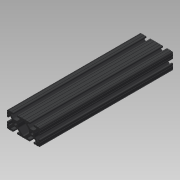
# Autodesk Inventor part: 1530
Saved by Autodesk Inventor 2013 (Build 170138000, 138)
## iProperties
Company: 80/20 Inc.
Created: 2014-04-23
Part Number: 1530
Material: Generic
Document SubType Name: Modeling
Density: 1 g/cm^3
Vendor: 80/20 Inc.
Engineer: Ross Bowman
Designer: Ross Bowman
Catalog Web Link: 8020.net
Material: 6105-T5 Aluminum
Author: Ross Bowman
Keywords: 80/20 , 8020 , T-Slot , Extrusion
Autodesk Inventor part; units mm, degrees
ref_plane "YZ Plane" through (0, 0, 0) normal (1, 0, 0) x (0, 1, 0)
ref_plane "XZ Plane" through (0, 0, 0) normal (0, 1, 0) x (-1, 0, 0)
ref_plane "XY Plane" through (0, 0, 0) normal (0, 0, 1) x (1, 0, 0)
sketch "Sketch1" plane through (0, 0, 0) normal (0, 0, 1) x (1, 0, 0)
  circle A0 centre (-19.05, 0) radius 3.3274
  circle A1 centre (19.05, 0) radius 3.3274
  arc A2 (0, -15.1131) -> (2.077, -14.2576) centre (0.0116, -12.1921) ccw
  arc A3 (-2.077, -14.2576) -> (0, -15.1131) centre (-0.0116, -12.1921) ccw
  line L0 (-10.9024, -5.4321) -> (-2.077, -14.2576)
  arc A4 (-12.2936, -2.0735) -> (-10.9024, -5.4321) centre (-7.5438, -2.0735) ccw
  line L1 (-12.2936, 2.0735) -> (-12.2936, -2.0735)
  arc A5 (-10.9024, 5.4321) -> (-12.2936, 2.0735) centre (-7.5438, 2.0735) ccw
  line L2 (-2.077, 14.2576) -> (-10.9024, 5.4321)
  arc A6 (0, 15.1131) -> (-2.077, 14.2576) centre (-0.0116, 12.1921) ccw
  arc A7 (2.077, 14.2576) -> (0, 15.1131) centre (0.0116, 12.1921) ccw
  line L3 (10.9024, 5.4321) -> (2.077, 14.2576)
  arc A8 (12.2936, 2.0735) -> (10.9024, 5.4321) centre (7.5438, 2.0735) ccw
  line L4 (12.2936, -2.0735) -> (12.2936, 2.0735)
  arc A9 (10.9024, -5.4321) -> (12.2936, -2.0735) centre (7.5438, -2.0735) ccw
  line L5 (2.077, -14.2576) -> (10.9024, -5.4321)
  arc A10 (8.9158, 13.5344) -> (9.1761, 12.9058) centre (9.8048, 13.5344) ccw
  line L6 (8.9158, 13.5344) -> (8.9158, 14.097)
  arc A11 (9.8048, 14.986) -> (8.9158, 14.097) centre (9.8048, 14.097) ccw
  line L7 (9.8048, 14.986) -> (13.4112, 14.986)
  arc A12 (13.4112, 14.986) -> (14.986, 16.5608) centre (13.4112, 16.5608) ccw
  line L8 (14.986, 16.5608) -> (14.986, 17.4968)
  arc A13 (14.986, 17.4968) -> (13.4328, 19.05) centre (13.4328, 17.4968) ccw
  line L9 (13.4328, 19.05) -> (10.9975, 19.05)
  arc A14 (9.4735, 19.05) -> (10.9975, 19.05) centre (10.2355, 19.05) ccw
  line L10 (9.4735, 19.05) -> (4.6451, 19.05)
  arc A15 (3.1211, 19.05) -> (4.6451, 19.05) centre (3.8831, 19.05) ccw
  line L11 (3.1211, 19.05) -> (-3.1211, 19.05)
  arc A16 (-4.6451, 19.05) -> (-3.1211, 19.05) centre (-3.8831, 19.05) ccw
  line L12 (-4.6451, 19.05) -> (-9.4735, 19.05)
  arc A17 (-10.9975, 19.05) -> (-9.4735, 19.05) centre (-10.2355, 19.05) ccw
  line L13 (-10.9975, 19.05) -> (-13.4328, 19.05)
  arc A18 (-13.4328, 19.05) -> (-14.986, 17.4968) centre (-13.4328, 17.4968) ccw
  line L14 (-14.986, 17.4968) -> (-14.986, 16.5608)
  arc A19 (-14.986, 16.5608) -> (-13.4112, 14.986) centre (-13.4112, 16.5608) ccw
  line L15 (-13.4112, 14.986) -> (-9.8048, 14.986)
  arc A20 (-8.9158, 14.097) -> (-9.8048, 14.986) centre (-9.8048, 14.097) ccw
  line L16 (-8.9158, 14.097) -> (-8.9158, 13.5344)
  arc A21 (-9.1761, 12.9058) -> (-8.9158, 13.5344) centre (-9.8048, 13.5344) ccw
  line L17 (-9.1761, 12.9058) -> (-13.8525, 8.2294)
  arc A22 (-17.2111, 6.8382) -> (-13.8525, 8.2294) centre (-17.2111, 11.588) ccw
  line L18 (-17.2111, 6.8382) -> (-20.8889, 6.8382)
  arc A23 (-24.2475, 8.2294) -> (-20.8889, 6.8382) centre (-20.8889, 11.588) ccw
  line L19 (-24.2475, 8.2294) -> (-28.9239, 12.9058)
  arc A24 (-29.1842, 13.5344) -> (-28.9239, 12.9058) centre (-28.2952, 13.5344) ccw
  line L20 (-29.1842, 13.5344) -> (-29.1842, 14.097)
  arc A25 (-28.2952, 14.986) -> (-29.1842, 14.097) centre (-28.2952, 14.097) ccw
  line L21 (-28.2952, 14.986) -> (-24.6888, 14.986)
  arc A26 (-24.6888, 14.986) -> (-23.114, 16.5608) centre (-24.6888, 16.5608) ccw
  line L22 (-23.114, 16.5608) -> (-23.114, 17.4806)
  arc A27 (-23.114, 17.4806) -> (-24.5589, 19.05) centre (-24.6888, 17.4806) ccw
  line L23 (-24.5589, 19.05) -> (-26.9458, 19.05)
  arc A28 (-28.4698, 19.05) -> (-26.9458, 19.05) centre (-27.7078, 19.05) ccw
  line L24 (-28.4698, 19.05) -> (-33.2963, 19.05)
  arc A29 (-34.8195, 19.0968) -> (-33.2963, 19.05) centre (-34.0579, 19.0734) ccw
  arc A30 (-34.8195, 19.0968) -> (-38.1376, 15.8983) centre (-34.903, 15.8631) ccw
  arc A31 (-38.1, 14.3752) -> (-38.1376, 15.8983) centre (-38.1, 15.1372) ccw
  line L25 (-38.1, 14.3752) -> (-38.1, 9.5497)
  arc A32 (-38.1, 8.0257) -> (-38.1, 9.5497) centre (-38.1, 8.7877) ccw
  line L26 (-38.1, 8.0257) -> (-38.1, 5.6388)
  arc A33 (-38.1, 5.6388) -> (-36.5252, 4.064) centre (-36.5252, 5.6388) ccw
  line L27 (-36.5252, 4.064) -> (-35.6108, 4.064)
  arc A34 (-35.6108, 4.064) -> (-34.036, 5.6388) centre (-35.6108, 5.6388) ccw
  line L28 (-34.036, 5.6388) -> (-34.036, 9.398)
  arc A35 (-33.147, 10.287) -> (-34.036, 9.398) centre (-33.147, 9.398) ccw
  line L29 (-33.147, 10.287) -> (-32.4207, 10.287)
  arc A36 (-31.792, 10.0266) -> (-32.4207, 10.287) centre (-32.4207, 9.398) ccw
  line L30 (-31.792, 10.0266) -> (-27.1976, 5.4321)
  arc A37 (-25.8064, 2.0735) -> (-27.1976, 5.4321) centre (-30.5562, 2.0735) ccw
  line L31 (-25.8064, 2.0735) -> (-25.8064, -2.0735)
  arc A38 (-27.1976, -5.4321) -> (-25.8064, -2.0735) centre (-30.5562, -2.0735) ccw
  line L32 (-27.1976, -5.4321) -> (-31.792, -10.0266)
  arc A39 (-32.4207, -10.287) -> (-31.792, -10.0266) centre (-32.4207, -9.398) ccw
  line L33 (-32.4207, -10.287) -> (-33.147, -10.287)
  arc A40 (-34.036, -9.398) -> (-33.147, -10.287) centre (-33.147, -9.398) ccw
  line L34 (-34.036, -9.398) -> (-34.036, -5.6388)
  arc A41 (-34.036, -5.6388) -> (-35.6108, -4.064) centre (-35.6108, -5.6388) ccw
  line L35 (-35.6108, -4.064) -> (-36.5252, -4.064)
  arc A42 (-36.5252, -4.064) -> (-38.1, -5.6388) centre (-36.5252, -5.6388) ccw
  line L36 (-38.1, -5.6388) -> (-38.1, -8.0257)
  arc A43 (-38.1, -9.5497) -> (-38.1, -8.0257) centre (-38.1, -8.7877) ccw
  line L37 (-38.1, -9.5497) -> (-38.1, -15.036)
  arc A44 (-38.1, -16.56) -> (-38.1, -15.036) centre (-38.1, -15.798) ccw
  arc A45 (-38.1, -16.56) -> (-35.5713, -19.05) centre (-34.9455, -15.8855) ccw
  arc A46 (-34.0473, -19.05) -> (-35.5713, -19.05) centre (-34.8093, -19.05) ccw
  line L38 (-34.0473, -19.05) -> (-28.4698, -19.05)
  arc A47 (-26.9458, -19.05) -> (-28.4698, -19.05) centre (-27.7078, -19.05) ccw
  line L39 (-26.9458, -19.05) -> (-24.6888, -19.05)
  arc A48 (-24.6888, -19.05) -> (-23.114, -17.4752) centre (-24.6888, -17.4752) ccw
  line L40 (-23.114, -17.4752) -> (-23.114, -16.5608)
  arc A49 (-23.114, -16.5608) -> (-24.6888, -14.986) centre (-24.6888, -16.5608) ccw
  line L41 (-24.6888, -14.986) -> (-28.448, -14.986)
  arc A50 (-29.337, -14.097) -> (-28.448, -14.986) centre (-28.448, -14.097) ccw
  line L42 (-29.337, -14.097) -> (-29.337, -13.6872)
  arc A51 (-29.0766, -13.0586) -> (-29.337, -13.6872) centre (-28.448, -13.6872) ccw
  line L43 (-29.0766, -13.0586) -> (-24.2475, -8.2294)
  arc A52 (-20.8889, -6.8382) -> (-24.2475, -8.2294) centre (-20.8889, -11.588) ccw
  line L44 (-20.8889, -6.8382) -> (-17.2111, -6.8382)
  arc A53 (-13.8525, -8.2294) -> (-17.2111, -6.8382) centre (-17.2111, -11.588) ccw
  line L45 (-13.8525, -8.2294) -> (-9.0234, -13.0586)
  arc A54 (-8.763, -13.6872) -> (-9.0234, -13.0586) centre (-9.652, -13.6872) ccw
  line L46 (-8.763, -13.6872) -> (-8.763, -14.097)
  arc A55 (-9.652, -14.986) -> (-8.763, -14.097) centre (-9.652, -14.097) ccw
  line L47 (-9.652, -14.986) -> (-13.4112, -14.986)
  arc A56 (-13.4112, -14.986) -> (-14.986, -16.5608) centre (-13.4112, -16.5608) ccw
  line L48 (-14.986, -16.5608) -> (-14.986, -17.4752)
  arc A57 (-14.986, -17.4752) -> (-13.4112, -19.05) centre (-13.4112, -17.4752) ccw
  line L49 (-13.4112, -19.05) -> (-10.9975, -19.05)
  arc A58 (-9.4735, -19.05) -> (-10.9975, -19.05) centre (-10.2355, -19.05) ccw
  line L50 (-9.4735, -19.05) -> (-4.6451, -19.05)
  arc A59 (-3.1211, -19.05) -> (-4.6451, -19.05) centre (-3.8831, -19.05) ccw
  line L51 (-3.1211, -19.05) -> (3.1211, -19.05)
  arc A60 (4.6451, -19.05) -> (3.1211, -19.05) centre (3.8831, -19.05) ccw
  line L52 (4.6451, -19.05) -> (9.4735, -19.05)
  arc A61 (10.9975, -19.05) -> (9.4735, -19.05) centre (10.2355, -19.05) ccw
  line L53 (10.9975, -19.05) -> (13.4112, -19.05)
  arc A62 (13.4112, -19.05) -> (14.986, -17.4752) centre (13.4112, -17.4752) ccw
  line L54 (14.986, -17.4752) -> (14.986, -16.5608)
  arc A63 (14.986, -16.5608) -> (13.4112, -14.986) centre (13.4112, -16.5608) ccw
  line L55 (13.4112, -14.986) -> (9.652, -14.986)
  arc A64 (8.763, -14.097) -> (9.652, -14.986) centre (9.652, -14.097) ccw
  line L56 (8.763, -14.097) -> (8.763, -13.6872)
  arc A65 (9.0234, -13.0586) -> (8.763, -13.6872) centre (9.652, -13.6872) ccw
  line L57 (9.0234, -13.0586) -> (13.8525, -8.2294)
  arc A66 (17.2111, -6.8382) -> (13.8525, -8.2294) centre (17.2111, -11.588) ccw
  line L58 (17.2111, -6.8382) -> (20.8889, -6.8382)
  arc A67 (24.2475, -8.2294) -> (20.8889, -6.8382) centre (20.8889, -11.588) ccw
  line L59 (24.2475, -8.2294) -> (29.0766, -13.0586)
  arc A68 (29.337, -13.6872) -> (29.0766, -13.0586) centre (28.448, -13.6872) ccw
  line L60 (29.337, -13.6872) -> (29.337, -14.097)
  arc A69 (28.448, -14.986) -> (29.337, -14.097) centre (28.448, -14.097) ccw
  line L61 (28.448, -14.986) -> (24.6888, -14.986)
  arc A70 (24.6888, -14.986) -> (23.114, -16.5608) centre (24.6888, -16.5608) ccw
  line L62 (23.114, -16.5608) -> (23.114, -17.4752)
  arc A71 (23.114, -17.4752) -> (24.6888, -19.05) centre (24.6888, -17.4752) ccw
  line L63 (24.6888, -19.05) -> (26.9458, -19.05)
  arc A72 (28.4698, -19.05) -> (26.9458, -19.05) centre (27.7078, -19.05) ccw
  line L64 (28.4698, -19.05) -> (34.0473, -19.05)
  arc A73 (35.5713, -19.05) -> (34.0473, -19.05) centre (34.8093, -19.05) ccw
  arc A74 (35.5713, -19.05) -> (38.1, -16.56) centre (34.9379, -15.8778) ccw
  arc A75 (38.1, -15.036) -> (38.1, -16.56) centre (38.1, -15.798) ccw
  line L65 (38.1, -15.036) -> (38.1, -9.5497)
  arc A76 (38.1, -8.0257) -> (38.1, -9.5497) centre (38.1, -8.7877) ccw
  line L66 (38.1, -8.0257) -> (38.1, -5.6388)
  arc A77 (38.1, -5.6388) -> (36.5252, -4.064) centre (36.5252, -5.6388) ccw
  line L67 (36.5252, -4.064) -> (35.6108, -4.064)
  arc A78 (35.6108, -4.064) -> (34.036, -5.6388) centre (35.6108, -5.6388) ccw
  line L68 (34.036, -5.6388) -> (34.036, -9.398)
  arc A79 (33.147, -10.287) -> (34.036, -9.398) centre (33.147, -9.398) ccw
  line L69 (33.147, -10.287) -> (32.4207, -10.287)
  arc A80 (31.792, -10.0266) -> (32.4207, -10.287) centre (32.4207, -9.398) ccw
  line L70 (31.792, -10.0266) -> (27.1976, -5.4321)
  arc A81 (25.8064, -2.0735) -> (27.1976, -5.4321) centre (30.5562, -2.0735) ccw
  line L71 (25.8064, -2.0735) -> (25.8064, 2.0735)
  arc A82 (27.1976, 5.4321) -> (25.8064, 2.0735) centre (30.5562, 2.0735) ccw
  line L72 (27.1976, 5.4321) -> (31.792, 10.0266)
  arc A83 (32.4207, 10.287) -> (31.792, 10.0266) centre (32.4207, 9.398) ccw
  line L73 (32.4207, 10.287) -> (33.147, 10.287)
  arc A84 (34.036, 9.398) -> (33.147, 10.287) centre (33.147, 9.398) ccw
  line L74 (34.036, 9.398) -> (34.036, 5.6388)
  arc A85 (34.036, 5.6388) -> (35.6108, 4.064) centre (35.6108, 5.6388) ccw
  line L75 (35.6108, 4.064) -> (36.5252, 4.064)
  arc A86 (36.5252, 4.064) -> (38.1, 5.6388) centre (36.5252, 5.6388) ccw
  line L76 (38.1, 5.6388) -> (38.1, 8.0257)
  arc A87 (38.1, 9.5497) -> (38.1, 8.0257) centre (38.1, 8.7877) ccw
  line L77 (38.1, 9.5497) -> (38.1, 14.3752)
  arc A88 (38.1376, 15.8983) -> (38.1, 14.3752) centre (38.1, 15.1372) ccw
  arc A89 (38.1376, 15.8983) -> (34.8195, 19.0968) centre (34.903, 15.8631) ccw
  arc A90 (33.2963, 19.05) -> (34.8195, 19.0968) centre (34.0579, 19.0734) ccw
  line L78 (33.2963, 19.05) -> (28.4698, 19.05)
  arc A91 (26.9458, 19.05) -> (28.4698, 19.05) centre (27.7078, 19.05) ccw
  line L79 (26.9458, 19.05) -> (24.5589, 19.05)
  arc A92 (24.5589, 19.05) -> (23.114, 17.4806) centre (24.6888, 17.4806) ccw
  line L80 (23.114, 17.4806) -> (23.114, 16.5608)
  arc A93 (23.114, 16.5608) -> (24.6888, 14.986) centre (24.6888, 16.5608) ccw
  line L81 (24.6888, 14.986) -> (28.2952, 14.986)
  arc A94 (29.1842, 14.097) -> (28.2952, 14.986) centre (28.2952, 14.097) ccw
  line L82 (29.1842, 14.097) -> (29.1842, 13.5344)
  arc A95 (28.9239, 12.9058) -> (29.1842, 13.5344) centre (28.2952, 13.5344) ccw
  line L83 (28.9239, 12.9058) -> (24.2475, 8.2294)
  arc A96 (20.8889, 6.8382) -> (24.2475, 8.2294) centre (20.8889, 11.588) ccw
  line L84 (20.8889, 6.8382) -> (17.2111, 6.8382)
  arc A97 (13.8525, 8.2294) -> (17.2111, 6.8382) centre (17.2111, 11.588) ccw
  line L85 (13.8525, 8.2294) -> (9.1761, 12.9058)
  point P0 (0, 0)
  constraints: 192 point on circle, 172 end point, 98 centre point
extrude "Extrusion1" add sketch "Sketch1" against normal blind 304.8
body "Solid1"
